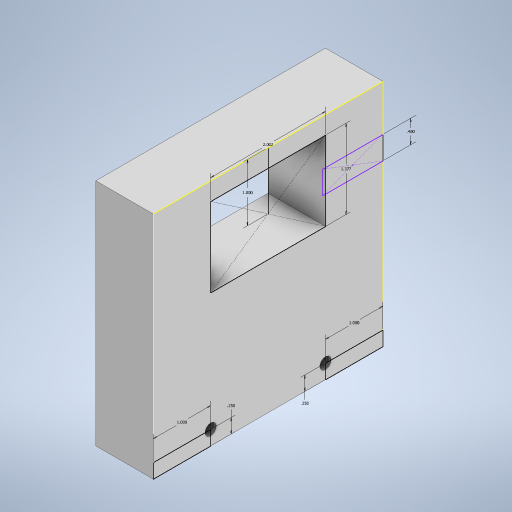
# Autodesk Inventor part: Al thermal core
Saved by Autodesk Inventor 2024.1 (Build 281209000, 209)
## iProperties
Created: 2024-08-21
Part Number: Al thermal core
Material: Generic
Document SubType Name: Modeling
Designer: pab2
Density: 1 g/cm^3
Appearance: Default
Author: pab2
Autodesk Inventor part; units mm, degrees
ref_plane "YZ Plane" through (0, 0, 0) normal (1, 0, 0) x (0, 1, 0)
ref_plane "XZ Plane" through (0, 0, 0) normal (0, 1, 0) x (-1, 0, 0)
ref_plane "XY Plane" through (0, 0, 0) normal (0, 0, 1) x (1, 0, 0)
sketch "Sketch1" plane through (0, 0, 0) normal (1, 0, 0) x (0, 1, 0)
  line L0 (0, 0) -> (101.6, 0)
  line L1 (101.6, 0) -> (101.6, -101.6)
  line L2 (101.6, -101.6) -> (0, -101.6)
  line L3 (0, -101.6) -> (0, 0)
  dimension "d0" = 101.6
  dimension "d1" = 101.6
  constraints: 8 end point, 2 parallel, 1 horizontal, 1 perpendicular
  measures "d0" distance of L1.end L2.end
  measures "d1" distance of L0.end L1.end
extrude "Extrusion1" add sketch "Sketch1" along normal blind 25.4
sketch "Sketch2" plane through (25.4, 0, 0) normal (1, 0, 0) x (0, 0, -1)
  line L0 (0, 101.6) -> (0, 0) projected
  line L1 (0, 0) -> (25.4, 0)
  line L2 (25.4, 0) -> (25.4, 6.35)
  line L3 (25.4, 6.35) -> (0, 6.35)
  line L4 (0, 6.35) -> (0, 0)
  line L5 (101.6, 0) -> (101.6, 101.6) projected
  line L6 (101.6, 0) -> (76.2, 0)
  line L7 (76.2, 0) -> (76.2, 6.35)
  line L8 (76.2, 6.35) -> (101.6, 6.35)
  line L9 (101.6, 6.35) -> (101.6, 0)
  line L10 (101.6, 101.6) -> (0, 101.6) projected
  line L11 (50.8, 101.6) -> (50.8, 76.2)
  line L12 (25.3746, 58.7121) -> (76.2254, 58.7121)
  line L13 (76.2254, 58.7121) -> (76.2254, 93.6879)
  line L14 (76.2254, 93.6879) -> (25.3746, 93.6879)
  line L15 (25.3746, 93.6879) -> (25.3746, 58.7121)
  line L16 (25.3746, 58.7121) -> (76.2254, 93.6879) construction
  line L17 (76.2254, 58.7121) -> (25.3746, 93.6879) construction
  line L18 (74.9076, 71.12) -> (101.6, 71.12)
  line L19 (101.6, 71.12) -> (101.6, 81.28)
  line L20 (101.6, 81.28) -> (74.9076, 81.28)
  line L21 (74.9076, 81.28) -> (74.9076, 71.12)
  line L22 (74.9076, 71.12) -> (101.6, 81.28) construction
  line L23 (101.6, 71.12) -> (74.9076, 81.28) construction
  point P0 (88.2538, 76.2)
  dimension "d4" = 25.4
  dimension "d5" = 6.35
  dimension "d6" = 25.4
  dimension "d7" = 6.35
  dimension "d8" = 25.4
  dimension "d9" = 50.8508
  dimension "d10" = 34.9758
  dimension "d20" = 10.16
  constraints: 42 end point, 8 parallel, 5 midpoint, 4 horizontal, 4 perpendicular, 1 point on line, 1 vertical
  measures "d4" distance of L3.end L2.end
  measures "d5" distance of L2.end L1.end
  measures "d6" distance of L7.end L8.end
  measures "d7" distance of L6.end L7.end
  measures "d8" distance of L11.start L11.end
  measures "d9" distance of L14.end L13.end
  measures "d10" distance of L13.end L12.end
  measures "d20" distance of L19.end L18.end
extrude "Extrusion2" cut sketch "Sketch2" against normal blind 25.4 contours L18 L21 L20 L13 | L13 L12 L15 L14 L20 L21 L18
hole "Hole1" at (25.4, 6.35, -76.2) at (25.4, 6.35, -25.4) direction (-1, 0, 0) diameter 4.9784 end through all thread size "1/4-20 UNC" class "2B" standard "ANSI Unified Screw Threads"
body "Solid1"
